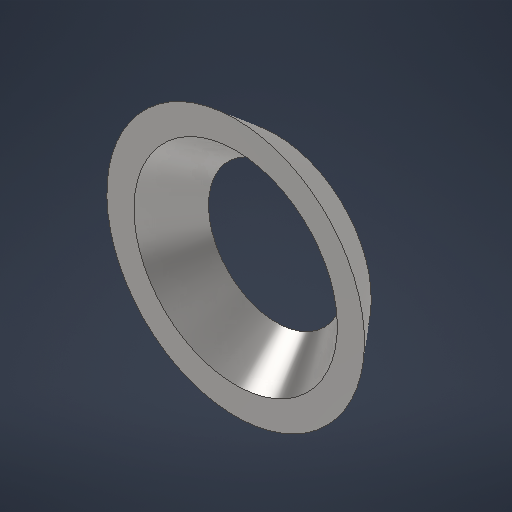
# Autodesk Inventor part: Collegamento2
Saved by Autodesk Inventor 2026.2 (Build 302298010, 298A)
## iProperties
Created: 2026-05-01
Part Number: Collegamento2
Material: Steel, Alloy
Document SubType Name: Modeling
Designer: Yan
Density: 7.73 g/cm^3
Appearance: Semi-Polished
Author: Yan
Autodesk Inventor part; units mm, degrees
ref_plane "YZ Plane" through (0, 0, 0) normal (1, 0, 0) x (0, 1, 0)
ref_plane "XZ Plane" through (0, 0, 0) normal (0, 1, 0) x (-1, 0, 0)
ref_plane "XY Plane" through (0, 0, 0) normal (0, 0, 1) x (1, 0, 0)
sketch "Sketch1" plane through (0, 0, 0) normal (1, 0, 0) x (0, 1, 0)
  line L0 (0, 0) -> (0, -30)
  line L1 (0, 0) -> (75, 0)
  line L2 (0, -30) -> (50, -30)
  line L3 (50, -30) -> (75, 0)
  line L4 (95, 0) -> (75, 0)
  line L5 (95, 0) -> (70, -30)
  line L6 (70, -30) -> (50, -30)
  dimension "d0" = 20
  dimension "d1" = 75
  dimension "d2" = 50
  dimension "d3" = 30
  constraints: 14 end point, 3 parallel, 2 horizontal, 1 point on line, 1 vertical
  measures "d0" distance of L4.start L1.end
  measures "d1" distance of L0.start L1.end
  measures "d2" distance of L0.end L2.end
  measures "d3" distance of L0.start L0.end
revolve "Revolution1" add sketch "Sketch1" angle 360 about axis through (0, 0, 0) along (0, 0, -1) contours L4 L5 L6 L3
body "Solid1"
